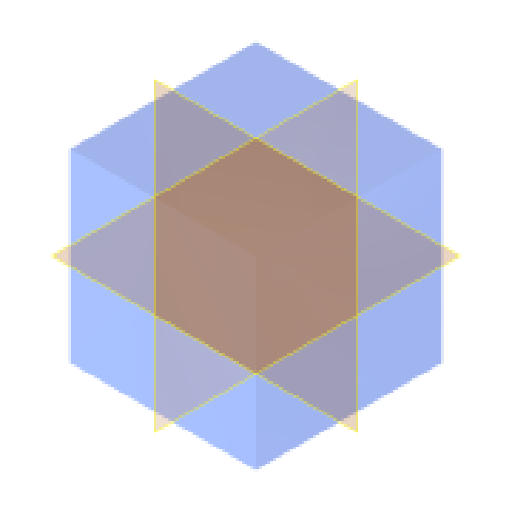
# Autodesk Inventor part: 00_Beamsplitter
Saved by Autodesk Inventor 2025.1 (Build 291241020, 241B)
## iProperties
Created: 2019-08-07
Part Number: 00_Beamsplitter
Material: Glass
Document SubType Name: Modeling
Designer: marsikovabarbora
Density: 2.18 g/cm^3
Appearance: Clear - Blue
Author: marsikovabarbora
Autodesk Inventor part; units mm, degrees
ref_plane "YZ Plane" through (0, 0, 0) normal (1, 0, 0) x (0, 1, 0)
ref_plane "XZ Plane" through (0, 0, 0) normal (0, 1, 0) x (-1, 0, 0)
ref_plane "XY Plane" through (0, 0, 0) normal (0, 0, 1) x (1, 0, 0)
sketch "Sketch1" plane through (0, 0, 0) normal (0, 0, 1) x (1, 0, 0)
  line L0 (-14, 0) -> (14, 0) construction
  line L1 (0, -14) -> (0, 14) construction
  line L2 (-10, 10) -> (10, 10)
  line L3 (10, 10) -> (10, -10)
  line L4 (10, -10) -> (-10, -10)
  line L5 (-10, -10) -> (-10, 10)
  point P0 (0, 0)
  dimension "d0" = 20
  dimension "d1" = 20
  constraints: 8 end point, 2 parallel, 1 horizontal, 1 perpendicular, 2 other
  measures "d0" distance of L2.start L2.end
  measures "d1" distance of L2.end L3.end
extrude "Extrusion1" add sketch "Sketch1" along normal blind 20
ref_plane "Work Plane1" through (0, -10, 0) normal (1, 0, 0) x (0, 0, -1)
ref_plane "Work Plane2" through (0, 0, 10) normal (0, 0, 1) x (1, 0, 0)
ref_plane "Work Plane3" through (-10, 0, 0) normal (0, 1, 0) x (1, 0, 0)
equation "\"d1\" = d0"
equation "\"d2\" = d0"
body "Solid1"
